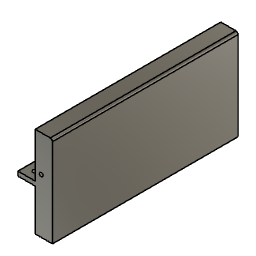
뒷 범퍼 (Autodesk Fusion 360 design; units mm, degrees)
Autodesk Fusion 360 part; units mm, degrees
sketch "스케치1" plane through (0, 0, 0) normal (0, 1, 0) x (1, 0, 0)
  line L0 (0, 0) -> (0, -105)
  line L1 (0, 0) -> (-3, 0)
  line L2 (-3, 0) -> (-3, -102)
  line L3 (-3, -102) -> (-20, -102)
  line L4 (0, -105) -> (-20, -105)
  line L5 (-20, -105) -> (-20, -102)
  dimension "d1" = 105
  dimension "d2" = 3
  dimension "d3" = 102
  dimension "d4" = 17
  constraint coincident L0.start L1.start
  constraint vertical L0
  constraint perpendicular L0 L1
  constraint perpendicular L1 L2
  constraint perpendicular L2 L3
  constraint perpendicular L0 L4
  measures "d1" distance of L0.start L0.end
  measures "d2" distance of L0.start L1.end
  measures "d3" distance of L1.end L2.end
  measures "d4" distance of L2.end L3.end
extrude "돌출1" add sketch "스케치1" along normal blind 215
sketch "스케치2" plane through (0, 0, 0) normal (0, -1, 0) x (1, 0, 0)
  line L0 (-3, 0) -> (0, 0)
  line L1 (0, 0) -> (0, 105)
  line L2 (0, 105) -> (-20, 105)
  line L3 (-20, 105) -> (-20, 102)
  line L4 (-20, 102) -> (-3, 102)
  line L5 (-3, 102) -> (-3, 0)
  line L6 (0, 105) -> (-20, 105)
  line L7 (-20, 105) -> (-20, 0)
  line L8 (-20, 0) -> (0, 0)
  line L9 (0, 0) -> (0, 105)
  line L10 (-3, 102) -> (-3, 73)
  line L11 (-3, 73) -> (-20, 73)
  line L12 (-20, 73) -> (-20, 53)
  line L13 (-20, 53) -> (-3, 53)
  line L14 (-3, 53) -> (-3, 73)
  line L15 (-20, 53) -> (-13, 53)
  line L16 (-13, 53) -> (-13, 63)
  line L17 (-13, 63) -> (-20, 63)
  line L18 (-20, 63) -> (-20, 53)
  circle A0 centre (-13, 63) radius 2.15
  dimension "d11" = 29
  dimension "d12" = 17
  dimension "d13" = 20
  dimension "d14" = 7
  dimension "d15" = 10
  dimension "d16" = 4.3
  constraint horizontal L6
  constraint vertical L7
  constraint horizontal L8
  constraint vertical L9
  constraint coincident L1.end L2.start
  constraint coincident L4.end L5.start
  constraint perpendicular L4 L10
  constraint horizontal L11
  constraint vertical L12
  constraint horizontal L13
  constraint vertical L14
  constraint horizontal L15
  constraint vertical L16
  constraint horizontal L17
  constraint vertical L18
  constraint coincident L16.end L17.start
  measures "d11" distance of L4.end L10.end
  measures "d12" distance of L10.end L11.end
  measures "d13" distance of L10.end L13.end
  measures "d14" distance of L12.end L15.end
  measures "d15" distance of L12.end L17.end
  measures "d16" diameter of A0
extrude "돌출2" add sketch "스케치2" against normal blind 3 contours L0 L1 L2 L3 L4 L5 L6 L7 L8 L9 L10 L14 | L5 L7 L8 L13 L15 | L5 L7 L11 L12 L13 L14 L16 L17 A0 | L4 L5 L7 L10 L11 | L7 L12 L13 L15 L16 L17 L18 A0
sketch "스케치3" plane through (0, 215, 0) normal (0, 1, 0) x (-1, 0, 0)
  line L0 (0, 0) -> (3, 0)
  line L1 (3, 0) -> (3, 102)
  line L2 (3, 102) -> (20, 102)
  line L3 (20, 102) -> (20, 105)
  line L4 (20, 105) -> (0, 105)
  line L5 (0, 105) -> (0, 0)
  line L6 (0, 105) -> (20, 105)
  line L7 (20, 105) -> (20, 0)
  line L8 (20, 0) -> (0, 0)
  line L9 (0, 0) -> (0, 105)
  line L10 (3, 102) -> (3, 73)
  line L11 (3, 73) -> (20, 73)
  line L12 (20, 73) -> (20, 53)
  line L13 (20, 53) -> (3, 53)
  line L14 (3, 53) -> (3, 73)
  line L15 (20, 53) -> (13, 53)
  line L16 (13, 53) -> (13, 63)
  line L17 (13, 63) -> (20, 63)
  line L18 (20, 63) -> (20, 53)
  circle A0 centre (13, 63) radius 2.15
  dimension "d17" = 29
  dimension "d18" = 17
  dimension "d19" = 20
  dimension "d20" = 7
  dimension "d21" = 10
  dimension "d22" = 4.3
  constraint horizontal L6
  constraint vertical L7
  constraint horizontal L8
  constraint vertical L9
  constraint coincident L4.end L5.start
  constraint coincident L1.end L2.start
  constraint perpendicular L2 L10
  constraint horizontal L11
  constraint vertical L12
  constraint horizontal L13
  constraint vertical L14
  constraint horizontal L15
  constraint vertical L16
  constraint horizontal L17
  constraint vertical L18
  constraint coincident L16.end L17.start
  measures "d17" distance of L1.end L10.end
  measures "d18" distance of L10.end L11.end
  measures "d19" distance of L10.end L13.end
  measures "d20" distance of L12.end L15.end
  measures "d21" distance of L12.end L17.end
  measures "d22" diameter of A0
extrude "돌출3" add sketch "스케치3" against normal blind 3 contours L1 L7 L8 L13 L15 | L1 L7 L11 L12 L13 L14 L16 L17 A0 | L1 L2 L7 L10 L11 | L7 L12 L13 L15 L16 L17 L18 A0
sketch "스케치4" plane through (-3, 0, 0) normal (-1, 0, 0) x (0, -1, 0)
  line L0 (-212, 102) -> (-212, 0)
  line L1 (-212, 0) -> (-3, 0)
  line L2 (-3, 0) -> (-3, 102)
  line L3 (-3, 102) -> (-212, 102)
  line L4 (-212, 102) -> (-212, 53)
  line L5 (-212, 53) -> (-195, 53)
  line L6 (-195, 53) -> (-195, 48)
  line L7 (-195, 48) -> (-212, 48)
  line L8 (-212, 48) -> (-212, 53)
  line L9 (-3, 53) -> (-20, 53)
  line L10 (-20, 53) -> (-20, 48)
  line L11 (-20, 48) -> (-3, 48)
  line L12 (-3, 48) -> (-3, 53)
  line L13 (-195, 53) -> (-112.5, 53)
  line L14 (-112.5, 53) -> (-102.5, 53)
  line L15 (-102.5, 53) -> (-102.5, 48)
  line L16 (-102.5, 48) -> (-112.5, 48)
  line L17 (-112.5, 48) -> (-112.5, 53)
  dimension "d23" = 49
  dimension "d24" = 17
  dimension "d25" = 5
  dimension "d26" = 17
  dimension "d27" = 5
  dimension "d28" = 82.5
  dimension "d29" = 10
  dimension "d30" = 5
  constraint coincident L0.start L3.end
  constraint perpendicular L3 L4
  constraint horizontal L5
  constraint vertical L6
  constraint horizontal L7
  constraint vertical L8
  constraint horizontal L9
  constraint vertical L10
  constraint horizontal L11
  constraint vertical L12
  constraint coincident L2 L9.start
  constraint perpendicular L6 L13
  constraint horizontal L14
  constraint vertical L15
  constraint horizontal L16
  constraint vertical L17
  measures "d23" distance of L0.start L4.end
  measures "d24" distance of L4.end L5.end
  measures "d25" distance of L4.end L7.end
  measures "d26" distance of L9.start L9.end
  measures "d27" distance of L9.start L11.end
  measures "d28" distance of L5.end L13.end
  measures "d29" distance of L13.end L14.end
  measures "d30" distance of L13.end L16.end
extrude "돌출4" add sketch "스케치4" along normal blind 37 contours L0 L5 L6 L7 L8 | L2 L9 L10 L11 L12 | L14 L15 L16 L17
extrude "돌출5" add 1 faces at (-26.6667, 3, 49.6667) along direction (0, -1, 0) blind 3
extrude "돌출6" add 1 faces at (-33.3333, 212, 51.3333) along direction (0, 1, 0) blind 3
sketch "스케치5" plane through (0, 0, 53) normal (0, 0, 1) x (-1, 0, 0)
  line L0 (3, -102.5) -> (3, -112.5)
  line L1 (3, -112.5) -> (40, -112.5)
  line L2 (40, -112.5) -> (40, -102.5)
  line L3 (40, -102.5) -> (3, -102.5)
  line L4 (40, -102.5) -> (20, -102.5)
  line L5 (20, -102.5) -> (20, -112.5)
  line L6 (20, -112.5) -> (40, -112.5)
  line L7 (40, -112.5) -> (40, -102.5)
  circle A0 centre (30, -107.5) radius 2.65
  circle A1 centre (30, -205) radius 2.65
  circle A2 centre (30, -10) radius 2.65
  dimension "d37" = 20
  dimension "d43" = 5.3
  dimension "d49" = 5.3
  dimension "d50" = 5.3
  constraint horizontal L4
  constraint vertical L5
  constraint horizontal L6
  constraint vertical L7
  constraint coincident L2.end L3.start
  measures "d37" distance of L2.end L4.end
  measures "d43" diameter of A0
  measures "d49" diameter of A1
  measures "d50" diameter of A2
extrude "돌출7" cut sketch "스케치5" against normal blind 5 contours A0 | A1 | A2
fillet "필렛1" radius 2.5 1 edges at (0, 107.5, 105)
